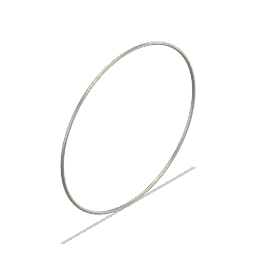
Double wheel design) (Autodesk Fusion 360 archive; units mm, degrees)
design "Roller Wire model"
Autodesk Fusion 360 part; units mm, degrees
sketch "Sketch1" plane through (0, 0, 0) normal (1, 0, 0) x (0, 0, -1)
  circle A0 centre (0, 0) radius 26
  dimension "d1" = 52
  constraint coincident A0.centre origin
  measures "d1" diameter of A0
pipe "Pipe1" add diameter 1 path "Sketch1" along A0
